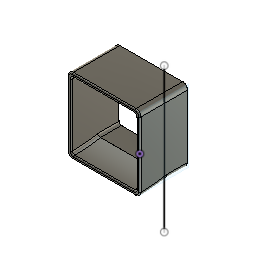
TAP-DIVERGE-REDUCED-V2 (Autodesk Fusion 360 design; units mm, degrees)
Autodesk Fusion 360 part; units mm, degrees
sketch "Sketch1" plane through (0, 0, 0) normal (0, 1, 0) x (1, 0, 0)
  line L0 (14.85, -14.85) -> (-14.85, -14.85)
  line L1 (-14.85, -14.85) -> (-14.85, 14.85)
  line L2 (-14.85, 14.85) -> (14.85, 14.85)
  line L3 (14.85, 14.85) -> (14.85, -14.85)
  line L4 (14.85, -14.85) -> (-14.85, 14.85) construction
  line L5 (-14.85, -14.85) -> (14.85, 14.85) construction
  dimension "d1" = 29.7
  dimension "d2" = 29.7
  constraint horizontal L0
  constraint perpendicular L0 L1
  constraint parallel L0 L2
  constraint parallel L1 L3
  constraint coincident L4 origin
  constraint coincident L5 origin
  measures "d1" distance of L1.end L2.end
  measures "d2" distance of L0.end L1.end
extrude "Extrude1" add sketch "Sketch1" along normal blind 20
sketch "Sketch2" plane through (0, 0, 0) normal (0, -1, 0) x (1, 0, 0)
  line L0 (-14.85, -14.85) -> (14.85, -14.85)
  line L1 (14.85, -14.85) -> (14.85, 14.85)
  line L2 (14.85, 14.85) -> (-14.85, 14.85)
  line L3 (-14.85, 14.85) -> (-14.85, -14.85)
  line L4 (13.25, -13.25) -> (-13.25, -13.25)
  line L5 (-13.25, -13.25) -> (-13.25, 13.25)
  line L6 (-13.25, 13.25) -> (13.25, 13.25)
  line L7 (13.25, 13.25) -> (13.25, -13.25)
  line L8 (13.25, -13.25) -> (-13.25, 13.25) construction
  line L9 (-13.25, -13.25) -> (13.25, 13.25) construction
  dimension "d5" = 26.5
  dimension "d6" = 26.5
  constraint horizontal L4
  constraint perpendicular L4 L5
  constraint parallel L4 L6
  constraint parallel L5 L7
  constraint coincident L8 origin
  constraint coincident L9 origin
  measures "d5" distance of L5.end L6.end
  measures "d6" distance of L4.end L5.end
extrude "Extrude2" cut sketch "Sketch2" against normal through all contours L4 L5 L6 L7
sketch "Sketch3" plane through (14.85, 0, 0) normal (1, 0, 0) x (0, 1, 0)
  line L0 (0, 14.85) -> (0, -14.85)
  line L1 (0, -14.85) -> (20, -14.85)
  line L2 (20, -14.85) -> (20, 14.85)
  line L3 (20, 14.85) -> (0, 14.85)
  line L4 (10, 26.2783) -> (10, -32.7983)
  dimension "d18" = 10
  constraint vertical L4
  measures "d18" distance of origin L4
sketch "Sketch4" plane through (14.85, 0, 0) normal (1, 0, 0) x (0, 1, 0)
sketch "Sketch5" plane through (14.85, 0, 0) normal (1, 0, 0) x (0, 1, 0)
  arc A0 (0, -15.8842) -> (11.2773, -14.85) centre (-0.3235, 49.6471) ccw
  line L0 (0, -15.8842) -> (0, -14.85)
  line L1 (0, -14.85) -> (11.2773, -14.85)
  constraint vertical L0
  constraint perpendicular L0 L1
extrude "Extrude3" add sketch "Sketch5" against normal blind 29.7
sketch "Sketch6" plane through (0, 0, 0) normal (0, -1, 0) x (1, 0, 0)
  line L0 (13.25, 13.25) -> (13.25, -13.25)
  line L1 (13.25, -13.25) -> (-13.25, -13.25)
  line L2 (-13.25, -13.25) -> (-13.25, 13.25)
  line L3 (-13.25, 13.25) -> (13.25, 13.25)
  line L4 (14.85, -15.8842) -> (14.85, 14.85)
  line L5 (14.85, 14.85) -> (-14.85, 14.85)
  line L6 (-14.85, 14.85) -> (-14.85, -15.8842)
  line L7 (-13.25, -13.25) -> (-13.25, -14.2842)
  line L8 (-13.25, -14.2842) -> (13.2442, -14.2842)
  line L9 (13.2442, -14.2842) -> (13.25, -13.25)
  line L10 (-14.85, -15.8842) -> (14.85, -15.8842)
  dimension "d10" = 1.95
  dimension "d27" = 1.6
  constraint coincident L1.end L2.start
  constraint perpendicular L1 L7
  constraint perpendicular L2 L8
  constraint coincident L0.end L1.start
  measures "d27" distance of L8 L10
sweep "Sweep1" cut profiles "Sketch6" along 1 edges at (14.85, 5.661, -15.6112) section 1 contours L1 L7 L8 L9
fillet "Fillet1" radius 2 6 edges at (-14.85, 10, 14.85) (14.85, 10, 14.85) (-14.85, 5.661, -15.6112) (14.85, 15.6386, -14.85) (14.85, 5.661, -15.6112) (-14.85, 15.6386, -14.85)
fillet "Fillet2" radius 1 6 edges at (-13.25, 10, 13.25) (13.25, 10, 13.25) (-13.25, 15.4988, -13.25) (13.25, 10, -13.25) (-13.25, 5.5228, -14.0171) (13.2442, 5.5228, -14.0171)
fillet "Fillet3" radius 0.5 16 edges at (-14.2642, 0, 14.2642) (-14.85, 0, -0.5171) (-14.2642, 0, -15.2984) (0, 0, -15.8842) (14.2642, 0, -15.2984) (14.85, 0, -0.5171) (14.2642, 0, 14.2642) (0, 0, 14.85) (12.9549, 0, -13.9933) (-0.0001, 0, -14.2842) (-12.9571, 0, -13.9913) (-13.25, 0, -0.5171) (-12.9571, 0, 12.9571) (0, 0, 13.25) (12.9571, 0, 12.9571) (13.25, 0, -0.5)
fillet "Fillet4" radius 0.5 16 edges at (14.2642, 20, 14.2642) (14.85, 20, 0) (14.2642, 20, -14.2642) (0, 20, -14.85) (-14.2642, 20, -14.2642) (-14.85, 20, 0) (-14.2642, 20, 14.2642) (0, 20, 14.85) (-12.9571, 20, 12.9571) (-13.25, 20, 0) (-12.9571, 20, -12.9571) (0, 20, -13.25) (12.9571, 20, -12.9571) (13.25, 20, 0) (12.9571, 20, 12.9571) (0, 20, 13.25)
